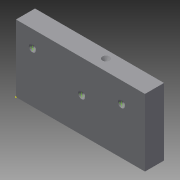
# Autodesk Inventor part: Part4
Saved by Autodesk Inventor 2015 (Build 190159000, 159)
## iProperties
Created: 2015-01-27
Part Number: Part4
Material: Generic
Document SubType Name: Modeling
Designer: PLTW-Stu-02
Density: 1 g/cm^3
Appearance: Default
Author: PLTW-Stu-02
Autodesk Inventor part; units mm, degrees
ref_plane "YZ Plane" through (0, 0, 0) normal (1, 0, 0) x (0, 1, 0)
ref_plane "XZ Plane" through (0, 0, 0) normal (0, 1, 0) x (-1, 0, 0)
ref_plane "XY Plane" through (0, 0, 0) normal (0, 0, 1) x (1, 0, 0)
sketch "Sketch1" plane through (0, 0, 0) normal (0, 0, 1) x (1, 0, 0)
  line L0 (0, 0) -> (171.9662, 0)
  line L1 (171.9662, 0) -> (171.9662, 89.5803)
  line L2 (171.9662, 89.5803) -> (0, 89.5803)
  line L3 (0, 89.5803) -> (0, 0)
  constraints: 8 end point, 2 parallel, 1 horizontal, 1 perpendicular
extrude "Extrusion1" add sketch "Sketch1" along normal blind 25.4
hole "Hole1" at (105.0559, 89.5803, 10.5119) direction (0, -1, 0) diameter 2.54 depth 9.525 tip angle 118 countersink diameter 9.525 countersink angle 82
sketch "Sketch2" plane through (0, 0, 25.4) normal (0, 0, 1) x (1, 0, 0)
  point P0 (0, 0)
sketch "Sketch3" plane through (0, 0, 25.4) normal (0, 0, 1) x (1, 0, 0)
  point P0 (0, 0)
  point P1 (21.8745, 67.3422)
  point P2 (140.6217, 62.3423)
  point P3 (87.498, 46.0927)
hole "Hole2" at (87.498, 46.0927, 25.4) at (140.6217, 62.3423, 25.4) at (21.8745, 67.3422, 25.4) direction (0, 0, -1) diameter 2.54 depth 9.525 tip angle 118 countersink diameter 9.525 countersink angle 82
body "Solid1"
